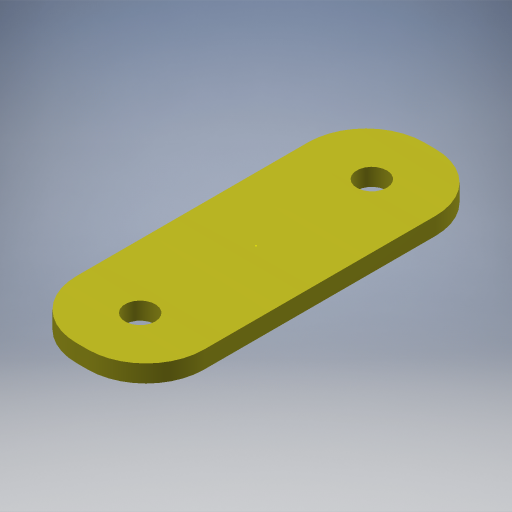
# Autodesk Inventor part: 24_0497_005
Saved by Autodesk Inventor 2024.3 (Build 283343000, 343)
## iProperties
Created: 2024-05-29
Part Number: 24_0497_005
Material: Allgemein
Document SubType Name: Modeling
Designer: Vogel
Density: 1 g/cm^3
Appearance: Kanariengelb
Author: Vogel
Autodesk Inventor part; units mm, degrees
ref_plane "YZ Plane" through (0, 0, 0) normal (1, 0, 0) x (0, 1, 0)
ref_plane "XZ Plane" through (0, 0, 0) normal (0, 1, 0) x (-1, 0, 0)
ref_plane "XY Plane" through (0, 0, 0) normal (0, 0, 1) x (1, 0, 0)
sketch "Skizze1" plane through (0, 0, 0) normal (0, 0, 1) x (1, 0, 0)
  line L0 (-15.4, 0) -> (15.4, 0) projected
  line L1 (0, -42) -> (0, 42) projected
  line L2 (11, -30) -> (-11, -30)
  line L3 (-11, -30) -> (-11, 30)
  line L4 (-11, 30) -> (11, 30)
  line L5 (11, 30) -> (11, -30)
  line L6 (11, -30) -> (-11, 30) construction
  line L7 (-11, -30) -> (11, 30) construction
  point P0 (0, 0)
  dimension "d0" = 60
  dimension "d1" = 22
  constraints: 12 end point, 2 midpoint, 2 parallel, 1 horizontal, 1 perpendicular
  measures "d0" distance of L2.end L3.end
  measures "d1" distance of L3.end L4.end
extrude "Extrusion1" add sketch "Skizze1" along normal blind 3
sketch "Skizze2" plane through (0, 0, 3) normal (0, 0, 1) x (1, 0, 0)
  line L0 (11, 30) -> (-11, 30) projected
  line L1 (-11, 30) -> (-11, -30) projected
  line L2 (-11, -30) -> (11, -30) projected
  line L3 (11, -30) -> (11, 30) projected
  line L4 (-17.5, 0) -> (17.5, 0) projected
  line L5 (0, -42) -> (0, 42) projected
  line L6 (3.1579, -20) -> (-3.1579, -20)
  line L7 (-3.1579, -20) -> (-3.1579, 20)
  line L8 (-3.1579, 20) -> (3.1579, 20)
  line L9 (3.1579, 20) -> (3.1579, -20)
  line L10 (3.1579, -20) -> (-3.1579, 20) construction
  line L11 (-3.1579, -20) -> (3.1579, 20) construction
  point P0 (0, 0)
  point P1 (0, 20)
  point P2 (0, -20)
  dimension "d4" = 40
  constraints: 12 end point, 4 midpoint, 2 parallel, 1 horizontal, 1 perpendicular
  measures "d4" distance of L6.end L7.end
hole "Bohrung1" at (0, 20, 3) at (0, -20, 3) direction (0, 0, -1) diameter 5.2 end through all
fillet "Rundung1" radius 10 4 edges at (-11, 30, 1.5) (11, 30, 1.5) (11, -30, 1.5) (-11, -30, 1.5)
sketch "Skizze3" plane through (0, 0, 3) normal (0, 0, 1) x (1, 0, 0)
  point P0 (0, 0)
